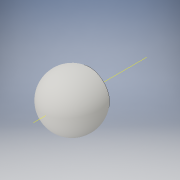
# Autodesk Inventor part: JS5210_hat_top_1
Saved by Autodesk Inventor 2016 (Build 200138000, 138)
## iProperties
Created: 2016-03-08
Part Number: JS5210_hat_top_1
Material: Generic
Document SubType Name: Modeling
Designer: twschum
Density: 1 g/cm^3
Appearance: Default
Author: twschum
Autodesk Inventor part; units mm, degrees
ref_plane "Work Plane1" through (0, 0, 0) normal (1, 0, 0) x (0, 0, -1)
sketch "Sketch3" plane through (0, 0, 0) normal (1, 0, 0) x (0, 0, -1)
  circle A0 centre (-3.3861, 0) radius 5.0734
  line L0 (-8.4595, 0) -> (1.6873, 0)
  line L1 (-0.0184, 0) -> (-0.0184, 3.7944)
  point P0 (0, 0)
  constraints: 4 end point, 3 point on circle, 1 centre point, 1 horizontal, 1 point on line, 1 vertical
ref_plane "Work Plane2" through (-0.85, -1.65, 0) normal (0, 0, 1) x (1, 0, 0)
sketch "Sketch5" plane through (-0.85, -1.65, 0) normal (0, 0, 1) x (1, 0, 0)
  line L0 (-0.8, 2.5) -> (0, 3.3) projected
  line L1 (-0.8, 0.8) -> (-0.8, 2.5) projected
  line L2 (0, 0) -> (-0.8, 0.8) projected
  line L3 (2.5, 0) -> (0, 0) projected
  line L4 (2.5, 3.3) -> (2.5, 0) projected
  line L5 (0, 3.3) -> (2.5, 3.3) projected
  circle A0 centre (0.85, 1.65) radius 1.25 projected
revolve "Revolution2" add sketch "Sketch3" angle 360 about axis through (0, 0, 8.4595) along (0, 0, -1) picked at (-5.6014, 0.385) contours L1 L0 A0
ref_plane "Work Plane3" through (-0.85, -1.65, 0) normal (0, 0, 1) x (1, 0, 0)
sketch "Sketch6" plane through (-0.85, -1.65, 0) normal (0, 0, 1) x (1, 0, 0)
  line L0 (0.85, 8.4832) -> (0.85, -5.1832) projected
  line L1 (-0.8, 2.5) -> (0, 3.3) projected
  line L2 (-0.8, 0.8) -> (-0.8, 2.5) projected
  line L3 (0, 0) -> (-0.8, 0.8) projected
  line L4 (2.5, 0) -> (0, 0) projected
  line L5 (2.5, 3.3) -> (2.5, 0) projected
  line L6 (0, 3.3) -> (2.5, 3.3) projected
  circle A0 centre (0.85, 1.65) radius 1.25 projected
  circle A1 centre (0.85, 1.65) radius 1.25 projected
extrude "Extrusion2" cut sketch "Sketch6" along normal blind 2.5
body "Solid1"
